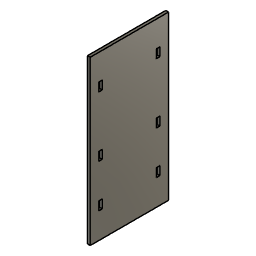
assembly v26 (Autodesk Fusion 360 archive; units mm, degrees)
design "electricalPanel"
Autodesk Fusion 360 part; units mm, degrees
sketch "Sketch1" plane through (0, 0, 0) normal (1, 0, 0) x (0, 1, 0)
  line L0 (0, 0) -> (45.6, 0)
  line L1 (45.6, 0) -> (45.6, 95)
  line L2 (45.6, 95) -> (0, 95)
  line L3 (0, 95) -> (0, 0)
  line L4 (5, 75) -> (7, 75)
  line L5 (7, 75) -> (7, 80)
  line L6 (7, 80) -> (5, 80)
  line L7 (5, 80) -> (5, 75)
  line L8 (38.6, 75) -> (40.6, 75)
  line L9 (40.6, 75) -> (40.6, 80)
  line L10 (40.6, 80) -> (38.6, 80)
  line L11 (38.6, 80) -> (38.6, 75)
  line L12 (5, 45) -> (7, 45)
  line L13 (7, 45) -> (7, 40)
  line L14 (7, 40) -> (5, 40)
  line L15 (5, 40) -> (5, 45)
  line L16 (38.6, 45) -> (40.6, 45)
  line L17 (40.6, 45) -> (40.6, 40)
  line L18 (40.6, 40) -> (38.6, 40)
  line L19 (38.6, 40) -> (38.6, 45)
  line L20 (5, 20) -> (7, 20)
  line L21 (7, 20) -> (7, 15)
  line L22 (7, 15) -> (5, 15)
  line L23 (5, 15) -> (5, 20)
  line L24 (38.6, 20) -> (40.6, 20)
  line L25 (40.6, 20) -> (40.6, 15)
  line L26 (40.6, 15) -> (38.6, 15)
  line L27 (38.6, 15) -> (38.6, 20)
  dimension "d1" = 45.6
  dimension "d2" = 95
  dimension "d3" = 2
  dimension "d4" = 2
  dimension "d5" = 5
  dimension "d6" = 5
  dimension "d7" = 5
  dimension "d8" = 15
  dimension "d9" = 30
  dimension "d10" = 15
  constraint horizontal L0
  constraint vertical L1
  constraint horizontal L2
  constraint vertical L3
  constraint coincident L0.start L3.end
  constraint horizontal L4
  constraint vertical L5
  constraint horizontal L6
  constraint vertical L7
  constraint horizontal L8
  constraint vertical L9
  constraint horizontal L10
  constraint vertical L11
  constraint horizontal L12
  constraint vertical L13
  constraint horizontal L14
  constraint vertical L15
  constraint horizontal L16
  constraint vertical L17
  constraint horizontal L18
  constraint vertical L19
  constraint horizontal L20
  constraint vertical L21
  constraint horizontal L22
  constraint vertical L23
  constraint horizontal L24
  constraint vertical L25
  constraint horizontal L26
  constraint vertical L27
  constraint vertical L13.end L20.end
  constraint vertical L5.end L12.end
  constraint vertical L10.end L16.start
  constraint vertical L18.end L24.start
  constraint vertical L17.end L24.end
  constraint vertical L9.end L16.end
  constraint vertical L6.end L12.start
  constraint vertical L14.end L20.start
  constraint horizontal L21.end L26.end
  constraint horizontal L20.end L24.start
  constraint horizontal L13.end L18.end
  constraint horizontal L12.end L16.start
  constraint horizontal L5.end L10.end
  constraint horizontal L4.end L8.start
  constraint equal L7 L15
  constraint equal L15 L23
  measures "d1" distance of L0.start L0.end
  measures "d2" distance of L0.start L2.end
  measures "d3" distance of L21.end L22.end
  measures "d4" distance of L25.end L26.end
  measures "d5" horizontal distance of L0.end L25.end
  measures "d6" horizontal distance of L0.start L22.end
  measures "d7" distance of L20.start L22.end
  measures "d8" vertical distance of L2.end L6.end
  measures "d9" distance of L4.start L12.start
  measures "d10" vertical distance of L0.start L22.end
extrude "Extrude1" add sketch "Sketch1" along normal blind 1.6

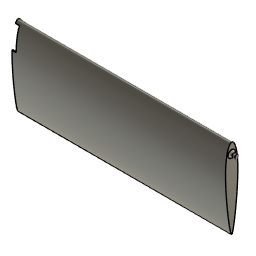
design "ailerons"
Autodesk Fusion 360 part; units mm, degrees
sketch "Sketch1" plane through (0, 0, 0) normal (1, 0, 0) x (0, 1, 0)
  spline S0 degree 5 poles (0, 0) (-0.0984, 0) (-0.2953, 0.2081) (-0.6031, 1.1448) (-1.0883, 3.5986) (-1.7768, 8.3639) (-2.4496, 14.3583) (-2.9457, 20.9396) (-3.1157, 27.3952) (-2.7821, 32.7537) (-2.0096, 36.5171) (-1.004, 38.6653) (0, 39.3389) (1.004, 38.6653) (2.0096, 36.5171) (2.7821, 32.7537) (3.1157, 27.3952) (2.9457, 20.9396) (2.4496, 14.3583) (1.7768, 8.3639) (1.0883, 3.5986) (0.6031, 1.1448) (0.2953, 0.2081) (0.0984, 0) (0, 0) knots 0 0 0 0 0 0 0.05 0.1 0.15 0.2 0.25 0.3 0.35 0.4 0.45 0.5 0.55 0.6 0.65 0.7 0.75 0.8 0.85 0.9 0.95 1 1 1 1 1 1
  line L0 (-3, 16) -> (-3, 36)
  line L1 (3, 36) -> (3, 16)
  line L2 (-1.5, 39) -> (1.5, 39)
  line L3 (0.5, 0) -> (-0.5, 0)
  point P0 (-3, 26)
  point P1 (0, 39)
  point P2 (3, 26)
  dimension "d1" = 26
  dimension "d2" = 13
  dimension "d4" = 6
  dimension "d5" = 20
  dimension "d6" = 1
  dimension "d7" = 3
  constraint coincident S0.start S0.end
  constraint midpoint P0 L0
  constraint vertical L0
  constraint midpoint P2 L1
  constraint vertical L1
  constraint midpoint P1 L2
  constraint horizontal L2
  constraint midpoint S0.start L3
  constraint horizontal L3
  constraint horizontal P0 P2
  constraint vertical S0.start P1
  constraint equal L0 L1
  measures "d1" distance of S0.start P0
  measures "d2" vertical distance of P0 P1
  measures "d4" distance of P0 P2
  measures "d5" distance of L1.start L1.end
  measures "d6" distance of L3.start L3.end
  measures "d7" distance of L2.start L2.end
extrude "Extrude1" add sketch "Sketch1" along normal blind 104
sketch "Sketch2" plane through (0, 0, 0) normal (-1, 0, 0) x (0, -1, 0)
  spline S0 degree 5 poles (0, 0) (0.0984, 0) (0.2953, 0.2081) (0.6031, 1.1448) (1.0883, 3.5986) (1.7768, 8.3639) (2.4496, 14.3583) (2.9457, 20.9396) (3.1157, 27.3952) (2.7821, 32.7537) (2.0096, 36.5171) (1.004, 38.6653) (0, 39.3389) (-1.004, 38.6653) (-2.0096, 36.5171) (-2.7821, 32.7537) (-3.1157, 27.3952) (-2.9457, 20.9396) (-2.4496, 14.3583) (-1.7768, 8.3639) (-1.0883, 3.5986) (-0.6031, 1.1448) (-0.2953, 0.2081) (-0.0984, 0) (0, 0) knots 0 0 0 0 0 0 0.05 0.1 0.15 0.2 0.25 0.3 0.35 0.4 0.45 0.5 0.55 0.6 0.65 0.7 0.75 0.8 0.85 0.9 0.95 1 1 1 1 1 1
  circle A0 centre (0, 34) radius 3.65
  circle A1 centre (0, 20) radius 2.25
  line L0 (2.2475, 19.8944) -> (2.8, 31.6585)
  line L1 (-2.2475, 19.8944) -> (-2.8, 31.6585)
  dimension "d10" = 7.3
  dimension "d11" = 4.5
  dimension "d12" = 14
  dimension "d13" = 5.6
  dimension "d14" = 34
  constraint coincident A1 L0.start
  constraint coincident A0 L0.end
  constraint coincident A1 L1.start
  constraint coincident A0 L1.end
  constraint vertical A0.centre A1.centre
  constraint vertical S0.start A1.centre
  constraint tangent A1 L1
  constraint tangent A1 L0
  constraint horizontal L0.end L1.end
  measures "d10" diameter of A0
  measures "d11" diameter of A1
  measures "d12" distance of A0.centre A1.centre
  measures "d13" horizontal distance of L0.end L1.end
  measures "d14" distance of S0.start A0.centre
extrude "Extrude2" cut sketch "Sketch2" against normal blind 2 contours S0 A0 A1 L0 L1 | S0 A0 | A1 picked at (0.1296, 33.0055)
sketch "Sketch3" plane through (104, 0, 0) normal (1, 0, 0) x (0, 1, 0)
  spline S0 degree 5 poles (0, 0) (0.0984, 0) (0.2953, 0.2081) (0.6031, 1.1448) (1.0883, 3.5986) (1.7768, 8.3639) (2.4496, 14.3583) (2.9457, 20.9396) (3.1157, 27.3952) (2.7821, 32.7537) (2.0096, 36.5171) (1.004, 38.6653) (0, 39.3389) (-1.004, 38.6653) (-2.0096, 36.5171) (-2.7821, 32.7537) (-3.1157, 27.3952) (-2.9457, 20.9396) (-2.4496, 14.3583) (-1.7768, 8.3639) (-1.0883, 3.5986) (-0.6031, 1.1448) (-0.2953, 0.2081) (-0.0984, 0) (0, 0) knots -1 -1 -1 -1 -1 -1 -0.95 -0.9 -0.85 -0.8 -0.75 -0.7 -0.65 -0.6 -0.55 -0.5 -0.45 -0.4 -0.35 -0.3 -0.25 -0.2 -0.15 -0.1 -0.05 0 0 0 0 0 0
  circle A0 centre (0, 34) radius 0.8
  dimension "d17" = 1.6
  dimension "d18" = 34
  constraint vertical S0.start A0.centre
  measures "d17" diameter of A0
  measures "d18" distance of S0.start A0.centre
extrude "Extrude3" add sketch "Sketch3" along normal blind 3 contours A0
fillet "Fillet1" radius 1 1 edges at (104, -0.7459, 34.2893)
fillet "Fillet1" radius 0.7 1 edges at (107, -0.7459, 33.7107)
fillet "Fillet1" radius 0.2 4 edges at (1, -1.5285, 37.3146) (1, 1.5285, 37.3146) (1, -2.7837, 31.3111) (1, 2.7837, 31.3111)

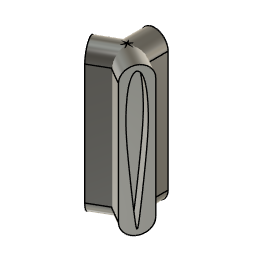
design "finHolder"
Autodesk Fusion 360 part; units mm, degrees
sketch "Sketch1" plane through (0, 0, 0) normal (0, 1, 0) x (1, 0, 0)
  line L0 (-5, 0) -> (5, 0)
  line L1 (5, 0) -> (5, -54)
  line L2 (5, -54) -> (-5, -54)
  line L3 (-5, -54) -> (-5, 0)
  dimension "d1" = 10
  dimension "d2" = 54
  dimension "d3" = 5
  constraint horizontal L0
  constraint vertical L1
  constraint horizontal L2
  constraint vertical L3
  constraint horizontal origin L0.end
  measures "d1" distance of L0.start L0.end
  measures "d2" distance of L0.start L2.end
  measures "d3" distance of origin L0.end
extrude "Extrude1" add sketch "Sketch1" along normal blind 10 makes body 1
sketch "Sketch2" plane through (0, 10, 0) normal (0, 1, 0) x (-1, 0, 0)
  line L0 (5, 54) -> (-5, 54)
  line L1 (-5, 54) -> (-5, 0)
  line L2 (-5, 0) -> (5, 0)
  line L3 (5, 0) -> (5, 54)
  spline S0 degree 5 poles (0, 2) (0.0829, 2) (0.2486, 2.4125) (0.5186, 4.2686) (1.0074, 8.9269) (1.7486, 16.855) (2.4545, 25.0304) (2.9459, 32.0654) (3.0612, 37.1221) (2.9371, 41.6893) (2.5475, 46.8402) (1.6202, 51.0987) (0, 52.8664) (-1.6202, 51.0987) (-2.5475, 46.8402) (-2.9371, 41.6893) (-3.0612, 37.1221) (-2.9459, 32.0654) (-2.4545, 25.0304) (-1.7486, 16.855) (-1.0074, 8.9269) (-0.5186, 4.2686) (-0.2486, 2.4125) (-0.0829, 2) (0, 2) knots 0 0 0 0 0 0 0.05 0.1 0.15 0.2 0.25 0.3 0.35 0.4 0.45 0.5 0.55 0.6 0.65 0.7 0.75 0.8 0.85 0.9 0.95 1 1 1 1 1 1
  line L4 (3, 32) -> (3, 42)
  line L5 (-3, 42) -> (-3, 32)
  line L6 (1.5, 52) -> (-1.5, 52)
  line L7 (-0.25, 2) -> (0.25, 2)
  point P0 (3, 37)
  point P1 (0, 52)
  point P2 (-3, 37)
  dimension "d13" = 35
  dimension "d14" = 15
  dimension "d15" = 0.5
  dimension "d16" = 3
  dimension "d17" = 10
  dimension "d18" = 6
  dimension "d19" = 3
  dimension "d20" = 2
  constraint horizontal P0 P2
  constraint midpoint P0 L4
  constraint vertical L4
  constraint midpoint P2 L5
  constraint vertical L5
  constraint midpoint P1 L6
  constraint horizontal L6
  constraint midpoint S0.start L7
  constraint horizontal L7
  constraint equal L4 L5
  constraint vertical origin S0.start
  constraint vertical origin P1
  measures "d13" distance of S0.start P2
  measures "d14" vertical distance of P1 P2
  measures "d15" distance of L7.start L7.end
  measures "d16" distance of L6.start L6.end
  measures "d17" distance of L4.start L4.end
  measures "d18" distance of P0 P2
  measures "d19" horizontal distance of P0 P1
  measures "d20" distance of origin S0.start
extrude "Extrude2" cut sketch "Sketch2" against normal blind 5 contours S0 bodies 1
pattern_circular "C-Pattern1" count 3 over 360 about axis through (0, 0, 1.75) along (0, 0, 1) of bodies 1 makes body 2 at (0.8333, -1.4434, 18) makes body 3 at (0.8333, 1.4434, 18)
fillet "Fillet1" radius 5 12 edges at (5, 5, 54) (-5, 5, 54) (5, 5, 0) (-5, 5, 0) (-6.8301, 1.8301, 54) (-1.8301, -6.8301, 54) (-1.8301, -6.8301, 0) (-6.8301, 1.8301, 0) (6.8301, 1.8301, 54) (1.8301, -6.8301, 54) (1.8301, -6.8301, 0) (6.8301, 1.8301, 0) on bodies 1 2 3

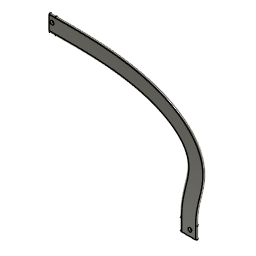
design "structuralThing"
Autodesk Fusion 360 part; units mm, degrees
sketch "Sketch1" plane through (0, 0, 0) normal (1, 0, 0) x (0, 1, 0)
  spline S0 degree 5 poles (0, 0) (0.1058, 0) (0.3174, 0.0986) (0.6269, 0.542) (0.9922, 1.6752) (1.3536, 3.7189) (1.6179, 6.0396) (1.7849, 8.3197) (1.8407, 10.3115) (1.7144, 12.0439) (1.3513, 13.4682) (0.7607, 14.426) (0, 14.7714) (-0.7607, 14.426) (-1.3513, 13.4682) (-1.7144, 12.0439) (-1.8407, 10.3115) (-1.7849, 8.3197) (-1.6179, 6.0396) (-1.3536, 3.7189) (-0.9922, 1.6752) (-0.6269, 0.542) (-0.3174, 0.0986) (-0.1058, 0) (0, 0) knots 0 0 0 0 0 0 0.05 0.1 0.15 0.2 0.25 0.3 0.35 0.4 0.45 0.5 0.55 0.6 0.65 0.7 0.75 0.8 0.85 0.9 0.95 1 1 1 1 1 1
  line L0 (1.8, 7.805) -> (1.8, 11.795)
  line L1 (-1.8, 11.795) -> (-1.8, 7.805)
  line L2 (0.74, 14.6) -> (-0.74, 14.6)
  line L3 (-0.345, 0) -> (0.345, 0)
  line L4 (0.8, 10.6) -> (0.8, 8.1)
  arc A0 (0.8, 8.1) -> (2.2, 8.1) centre (1.5, 8.1) ccw
  line L5 (2.2, 8.1) -> (2.2, 10.6)
  arc A1 (2.2, 10.6) -> (0.8, 10.6) centre (1.5, 10.6) ccw
  line L6 (1.5, 10.6) -> (1.5, 8.1) construction
  line L7 (-5.6108, 0) -> (-1, 0)
  line L8 (-1, 0) -> (-1, 14.6)
  line L9 (-1, 14.6) -> (-5.6108, 14.6)
  line L10 (-5.6108, 14.6) -> (-5.6108, 0)
  point P0 (1.8, 9.8)
  point P1 (0, 14.6)
  point P2 (-1.8, 9.8)
  dimension "d1" = 9.8
  dimension "d2" = 4.8
  dimension "d3" = 3.6
  dimension "d4" = 1.8
  dimension "d7" = 3.99
  dimension "d8" = 1.48
  dimension "d9" = 0.69
  dimension "d22" = 2.5
  dimension "d23" = 0.7
  dimension "d32" = 1.5
  dimension "d33" = 4
  dimension "d50" = 1
  constraint coincident S0.start S0.end
  constraint horizontal P0 P2
  constraint vertical S0.start P1
  constraint midpoint P0 L0
  constraint vertical L0
  constraint midpoint P2 L1
  constraint vertical L1
  constraint equal L0 L1
  constraint midpoint P1 L2
  constraint midpoint S0.start L3
  constraint horizontal L2
  constraint horizontal L3
  constraint tangent L4 A0
  constraint tangent A0 L5
  constraint parallel L4 L5
  constraint tangent L5 A1
  constraint tangent L4 A1
  constraint parallel L0 L6
  constraint horizontal L7
  constraint vertical L8
  constraint horizontal L9
  constraint vertical L10
  constraint horizontal S0.start L7.end
  constraint horizontal P1 L8.end
  measures "d1" distance of S0.start P2
  measures "d2" vertical distance of P1 P2
  measures "d3" distance of P0 P2
  measures "d4" horizontal distance of P0 P1
  measures "d7" distance of L0.start L0.end
  measures "d8" distance of L2.start L2.end
  measures "d9" distance of L3.start L3.end
  measures "d22" distance of A1.centre A0.centre
  measures "d23" radius of A1
  measures "d32" horizontal distance of P1 A1.centre
  measures "d33" vertical distance of P1 A1.centre
  measures "d50" distance of S0.start L7.end
sketch "Sketch2" plane through (0, 0, 0) normal (0, 1, 0) x (1, 0, 0)
  spline S0 degree 5 poles (0, 0) (2.3895, 0) (7.6554, -0.0112) (17.0138, -0.0623) (32.1264, 0.0249) (53.6486, 1.493) (75.4441, 5.5778) (94.6141, 12.9773) (108.4792, 23.7731) (113.5969, 35.5521) (111.6509, 47.8729) (108.0834, 59.0827) (106.3787, 68.8945) (106, 76.175) (106, 80) knots 0 0 0 0 0 0 0.1 0.2 0.3 0.4 0.5 0.6 0.7 0.8 0.9 1 1 1 1 1 1
  line L0 (106, 48.0702) -> (106, 111.9298)
  line L1 (-14.7723, 0) -> (14.7723, 0)
  line L2 (88.2721, 7.1271) -> (118.1197, 34.4401)
  point P0 (103.1959, 20.7836)
  dimension "d10" = 80
  dimension "d11" = 106
  constraint coincident S0.start origin
  constraint midpoint S0.end L0
  constraint vertical L0
  constraint midpoint S0.start L1
  constraint horizontal L1
  constraint midpoint P0 L2
  measures "d10" distance of S0.end S0.start
  measures "d11" distance of S0.start S0.end
sweep "Sweep1" add profiles "Sketch1" path "Sketch2" along S0 section 1 contours S0 L4 A0 A1 L8
extrude "Extrude2" add 1 faces at (0, -0.4, 7.9981) along direction (-1, 0, 0) blind 5
extrude "Extrude3" add 1 faces at (113.9981, -0.4, -80) along direction (0, 0, -1) blind 10
sketch "Sketch3" plane through (0, 0, 0) normal (0, 1, 0) x (1, 0, 0)
  circle A0 centre (-2.5, -9) radius 1.6
  circle A1 centre (115, 85) radius 1.6
  line L0 (106, 90) -> (113.4315, 90)
  line L1 (117.257, 90) -> (120.6, 90)
  dimension "d24" = 3.2
  dimension "d25" = 3.2
  dimension "d26" = 9
  dimension "d27" = 2.5
  dimension "d51" = 5
  dimension "d53" = 9
  measures "d24" diameter of A0
  measures "d25" diameter of A1
  measures "d26" vertical distance of origin A0.centre
  measures "d27" horizontal distance of origin A0.centre
  measures "d51" vertical distance of A1.centre L1.end
  measures "d53" horizontal distance of A1.centre L0.start
extrude "Extrude4" cut sketch "Sketch3" along normal mid plane 20
equation "d22 = 4 mm - 1.5 mm"
equation "d23 = ( 1.4 / 2 ) * 1 mm"
equation "d43 = 4 mm - 1.5 mm"
equation "d44 = ( 1.5 / 2 ) * 1 mm"
